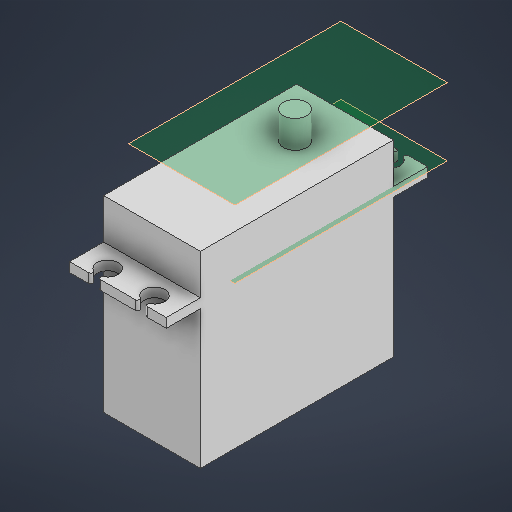
# Autodesk Inventor part: SM-S4303R
Saved by Autodesk Inventor 2025.2 (Build 292293000, 293)
## iProperties
Created: 2024-11-14
Part Number: SM-S4303R
Material: Generic
Document SubType Name: Modeling
Designer: JL
Density: 1 g/cm^3
Appearance: Default
Author: JL
Autodesk Inventor part; units mm, degrees
ref_plane "YZ Plane" through (0, 0, 0) normal (1, 0, 0) x (0, 1, 0)
ref_plane "XZ Plane" through (0, 0, 0) normal (0, 1, 0) x (-1, 0, 0)
ref_plane "XY Plane" through (0, 0, 0) normal (0, 0, 1) x (1, 0, 0)
sketch "Sketch1" plane through (0, 0, 0) normal (0, 1, 0) x (-1, 0, 0)
  line L0 (10.35, 0) -> (-10.35, 0)
  line L1 (-10.35, 0) -> (-10.35, 41.3)
  line L2 (-10.35, 41.3) -> (10.35, 41.3)
  line L3 (10.35, 41.3) -> (10.35, 0)
  point P0 (0, 0)
  point P1 (0, 0)
  dimension "d0" = 41.3
  dimension "d1" = 20.7
  constraints: 8 end point, 2 coincident, 2 parallel, 1 horizontal, 1 midpoint, 1 perpendicular
  measures "d0" distance of L0.end L1.end
  measures "d1" distance of L1.end L2.end
extrude "Extrusion1" add sketch "Sketch1" against normal blind 40.2
ref_plane "Work Plane2" through (0, -8.6, 0) normal (0, -1, 0) x (1, 0, 0)
ref_plane "Work Plane1" through (0, 5.9, 0) normal (0, -1, 0) x (1, 0, 0)
sketch "Sketch2" plane through (0, -8.6, 0) normal (0, -1, 0) x (1, 0, 0)
  line L0 (-10.35, 0) -> (10.35, 0) projected
  line L1 (-10.35, 41.3) -> (-10.35, 0) construction
  line L2 (-10.35, 0) -> (-10.35, -7.3)
  line L3 (-10.35, -7.3) -> (-6.25, -7.3)
  arc A0 (-6.25, -7.3) -> (-6.0496, -6.4902) centre (-6.25, -6.8703) ccw
  arc A1 (-3.9504, -6.4902) -> (-6.0496, -6.4902) centre (-5, -4.5) ccw
  arc A2 (-3.9504, -6.4902) -> (-3.75, -7.3) centre (-3.75, -6.8703) ccw
  line L4 (-3.75, -7.3) -> (0, -7.3)
  line L5 (0, -7.3) -> (0, 0) construction
  line L6 (10.35, 0) -> (10.35, -7.3)
  line L7 (10.35, -7.3) -> (6.25, -7.3)
  arc A3 (6.0496, -6.4902) -> (6.25, -7.3) centre (6.25, -6.8703) ccw
  arc A4 (6.0496, -6.4902) -> (3.9504, -6.4902) centre (5, -4.5) ccw
  arc A5 (3.75, -7.3) -> (3.9504, -6.4902) centre (3.75, -6.8703) ccw
  line L8 (3.75, -7.3) -> (0, -7.3)
  line L9 (-10.35, 20.65) -> (10.35, 20.65) construction
  line L10 (10.35, 0) -> (10.35, 41.3) construction
  line L11 (-10.35, 41.3) -> (10.35, 41.3)
  line L12 (-10.35, 41.3) -> (-10.35, 48.6)
  line L13 (-10.35, 48.6) -> (-6.25, 48.6)
  arc A6 (-6.0496, 47.7902) -> (-6.25, 48.6) centre (-6.25, 48.1703) ccw
  arc A7 (-6.0496, 47.7902) -> (-3.9504, 47.7902) centre (-5, 45.8) ccw
  arc A8 (-3.75, 48.6) -> (-3.9504, 47.7902) centre (-3.75, 48.1703) ccw
  line L14 (-3.75, 48.6) -> (0, 48.6)
  line L15 (0, 48.6) -> (0, 41.3) construction
  line L16 (10.35, 48.6) -> (6.25, 48.6)
  arc A9 (6.25, 48.6) -> (6.0496, 47.7902) centre (6.25, 48.1703) ccw
  arc A10 (3.9504, 47.7902) -> (6.0496, 47.7902) centre (5, 45.8) ccw
  arc A11 (3.9504, 47.7902) -> (3.75, 48.6) centre (3.75, 48.1703) ccw
  line L17 (3.75, 48.6) -> (0, 48.6)
  line L18 (10.35, 41.3) -> (10.35, 48.6)
  dimension "d7" = 4.5
  dimension "d8" = 10
  dimension "d9" = 55.9
  dimension "d10" = 50.3
  dimension "d11" = 2.5
  constraints: 32 end point, 26 symmetric about line, 24 point on circle, 12 centre point, 4 tangent, 3 midpoint, 2 horizontal, 1 collinear, 1 equal radius, 1 perpendicular, 1 vertical, 9 other
  measures "d7" diameter of A1
  measures "d8" distance of A4.centre A1.centre
  measures "d9" distance of L12.end L2.end
  measures "d10" distance of A1.centre A7.centre
  measures "d11" distance of A2.centre A0.centre
extrude "Extrusion2" add sketch "Sketch2" along normal blind 2
sketch "Sketch3" plane through (0, 5.9, 0) normal (0, -1, 0) x (1, 0, 0)
  circle A0 centre (0, 10.7) radius 2.5
  arc A1 (-3.9504, -6.4902) -> (-6.0496, -6.4902) centre (-5, -4.5) ccw construction
  point P0 (0, 0)
  dimension "d17" = 5
  dimension "d18" = 15.2
  constraints: 1 centre point, 1 vertical alignment
  measures "d17" diameter of A0
  measures "d18" vertical distance of A0.centre A1.centre
extrude "Extrusion3" add sketch "Sketch3" along normal up to next
body "Solid1"
